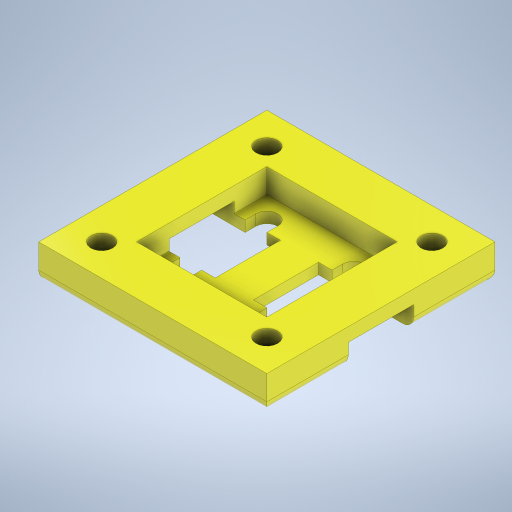
# Autodesk Inventor part: encoder_cover
Saved by Autodesk Inventor 2024 (Build 280153000, 153)
## iProperties
Created: 2021-10-17
Part Number: encoder_cover
Material: Generic
Document SubType Name: Modeling
Designer: jcgg2
Mass: 11.3449 g
Surface Area: 82.1762 cm^2
Volume: 11.3449 cm^3
Density: 1 g/cm^3
Appearance: Yellow
Author: jcgg2
Autodesk Inventor part; units mm, degrees
sketch "Sketch1" plane through (0, 0, 0) normal (0, 1, 0) x (-1, 0, 0)
  line L0 (21, 21) -> (-21, 21)
  line L1 (-21, 21) -> (-21, -21)
  line L2 (-21, -21) -> (21, -21)
  line L3 (21, -21) -> (21, 21)
  line L4 (21, 21) -> (-21, -21) construction
  line L5 (-21, 21) -> (21, -21) construction
  point P0 (0, 0)
  dimension "d0" = 42
  dimension "d1" = 42
  constraints: 12 end point, 2 midpoint, 2 parallel, 1 horizontal, 1 perpendicular
  measures "d0" distance of L2.end L1.end
  measures "d1" distance of L1.end L0.end
extrude "Extrusion1" add sketch "Sketch1" along normal blind 6.5
sketch "Sketch2" plane through (0, 6.5, 0) normal (0, 1, 0) x (1, 0, 0)
  line L0 (-12, -12) -> (12, -12)
  line L1 (12, -12) -> (12, 12)
  line L2 (12, 12) -> (-12, 12)
  line L3 (-12, 12) -> (-12, -12)
  line L4 (-12, -12) -> (12, 12) construction
  line L5 (12, -12) -> (-12, 12) construction
  point P0 (0, 0)
  dimension "d4" = 24
  dimension "d5" = 24
  constraints: 12 end point, 2 midpoint, 2 parallel, 1 horizontal, 1 perpendicular
  measures "d4" distance of L2.end L1.end
  measures "d5" distance of L1.end L0.end
extrude "Extrusion2" cut sketch "Sketch2" against normal blind 4.5
sketch "Sketch3" plane through (0, 2, 0) normal (0, 1, 0) x (1, 0, 0)
  line L0 (-10.5, -6) -> (-3.5, -6)
  line L1 (-3.5, -6) -> (-3.5, 6)
  line L2 (-3.5, 6) -> (-10.5, 6)
  line L3 (-10.5, 6) -> (-10.5, -6)
  line L4 (-10.5, -6) -> (-3.5, 6) construction
  line L5 (-3.5, -6) -> (-10.5, 6) construction
  line L6 (-12, -12) -> (-12, 12) projected
  line L7 (3.5, -6) -> (10.5, -6)
  line L8 (10.5, -6) -> (10.5, 6)
  line L9 (10.5, 6) -> (3.5, 6)
  line L10 (3.5, 6) -> (3.5, -6)
  line L11 (3.5, -6) -> (10.5, 6) construction
  line L12 (10.5, -6) -> (3.5, 6) construction
  line L13 (12, 12) -> (12, -12) projected
  point P0 (0, 0)
  point P1 (-7, 0)
  point P2 (-7, 0)
  point P3 (7, 0)
  point P4 (7, 0)
  dimension "d8" = 7
  dimension "d9" = 12
  dimension "d10" = 1.5
  dimension "d11" = 7
  dimension "d12" = 1.5
  dimension "d13" = 12
  constraints: 24 end point, 6 midpoint, 4 parallel, 2 horizontal, 2 horizontal alignment, 2 perpendicular
  measures "d8" distance of L2.end L1.end
  measures "d9" distance of L1.end L0.end
  measures "d10" distance between parallel lines of L6 L3
  measures "d11" distance of L9.end L8.end
  measures "d12" distance between parallel lines of L8 L13
  measures "d13" distance of L7.end L8.end
extrude "Extrusion3" cut sketch "Sketch3" against normal blind 3.5
sketch "Sketch4" plane through (0, 2, 0) normal (0, 1, 0) x (1, 0, 0)
  line L0 (-12, -12) -> (-12, 12) projected
  line L1 (12, -12) -> (-12, -12) projected
  point P0 (0, 0)
  point P1 (-8, -8)
  point P2 (-8, 8)
  point P3 (8, 8)
  point P4 (8, -8)
  dimension "d16" = 16
  dimension "d17" = 16
  dimension "d18" = 4
  dimension "d19" = 4
  constraints: 2 horizontal alignment, 2 vertical alignment
  measures "d16" distance of point (-8, -8) point (-8, 8)
  measures "d17" distance of point (-8, -8) point (8, -8)
  measures "d18" distance from line of L0 point (-8, -8)
  measures "d19" distance from line of L1 point (-8, -8)
hole "Hole1" at (-8, 2, 8) at (-8, 2, -8) at (8, 2, -8) at (8, 2, 8) direction (0, -1, 0) diameter 4 end through all
sketch "Sketch5" plane through (0, 6.5, 0) normal (0, 1, 0) x (1, 0, 0)
  line L0 (-21, -21) -> (21, -21) projected
  line L1 (-21, 21) -> (-21, -21) projected
  point P0 (0, 0)
  point P1 (-15.2, -15.2)
  point P2 (-15.2, 15.2)
  point P3 (15.2, 15.2)
  point P4 (15.2, -15.2)
  dimension "d27" = 30.4
  dimension "d28" = 30.4
  dimension "d29" = 5.8
  dimension "d30" = 5.8
  constraints: 2 horizontal alignment, 2 vertical alignment
  measures "d27" distance of point (-15.2, 15.2) point (-15.2, -15.2)
  measures "d28" distance of point (15.2, -15.2) point (-15.2, -15.2)
  measures "d29" distance from line of L0 point (-15.2, -15.2)
  measures "d30" distance from line of L1 point (-15.2, -15.2)
hole "Hole2" at (-15.2, 6.5, 15.2) at (-15.2, 6.5, -15.2) at (15.2, 6.5, -15.2) at (15.2, 6.5, 15.2) direction (0, -1, 0) diameter 4 end through all
ref_plane "Work Plane5" through (-25, 0, -21) normal (-1, 0, 0) x (0, 0, 1)
sketch "Sketch9" plane through (-25, 0, -21) normal (-1, 0, 0) x (0, 0, 1)
  point P0 (21, 0)
ref_plane "Work Plane4" through (25, 0, 21) normal (1, 0, 0) x (0, 0, -1)
sketch "Sketch10" plane through (25, 0, 21) normal (1, 0, 0) x (0, 0, -1)
  line L0 (27, 2) -> (31, 2) projected
  line L1 (27, 2) -> (15, 2) projected
  line L2 (11, 2) -> (15, 2) projected
  line L3 (15, 2) -> (27, 2) projected
  line L4 (27, 2) -> (31, 2) projected
  line L5 (27, 2) -> (15, 2) projected
  line L6 (11, 2) -> (15, 2) projected
  line L7 (15, 2) -> (27, 2) projected
  line L8 (33, 2) -> (9, 2) projected
  line L9 (9, 2) -> (33, 2) projected
  line L10 (27, 2) -> (15, 2) projected
  line L11 (27, 2) -> (27, 0) projected
  line L12 (15, 2) -> (27, 2) projected
  line L13 (15, 2) -> (15, 0) projected
  line L14 (27, 0) -> (15, 0) projected
  point P0 (21, 0)
  constraints: 1 other
extrude "Extrusion7" cut sketch "Sketch10" against normal blind 15
ref_plane "Work Plane6" through (-25, 0, -21) normal (-1, 0, 0) x (0, 0, 1)
sketch "Sketch11" plane through (-25, 0, -21) normal (-1, 0, 0) x (0, 0, 1)
  line L0 (27, 2) -> (27, 0) projected
  line L1 (15, 2) -> (27, 2) projected
  line L2 (15, 2) -> (15, 0) projected
  line L3 (27, 0) -> (15, 0) projected
  point P0 (21, 0)
extrude "Extrusion8" cut sketch "Sketch11" against normal blind 15
ref_plane "Work Plane7" through (-25, 0, 6) normal (-1, 0, 0) x (0, 0, 1)
ref_plane "Work Plane8" through (-25, 0, 6) normal (-1, 0, 0) x (0, 0, 1)
ref_plane "Work Plane9" through (-25, 2, -6) normal (0, -1, 0) x (1, 0, 0)
sketch "Sketch16" plane through (-25, 2, -6) normal (0, -1, 0) x (1, 0, 0)
  line L0 (13, 12) -> (13, 0) projected
  line L1 (4, 12) -> (13, 12) projected
  line L2 (4, 0) -> (13, 0) projected
  line L3 (37, 0) -> (37, 12) projected
  line L4 (50, 0) -> (37, 0) projected
  line L5 (50, 12) -> (50, 0) projected
  line L6 (50, 12) -> (37, 12) projected
  line L7 (4, 0) -> (4, 12) projected
  point P0 (25, 6)
extrude "Extrusion11" cut sketch "Sketch16" against normal blind 2
ref_plane "Work Plane10" through (-21, 6.5, 21) normal (1, 0, 0) x (0, 0, -1)
ref_plane "Work Plane11" through (-25, 0, 6) normal (-1, 0, 0) x (0, 0, 1)
fillet "Fillet4" radius 2 4 edges at (21, 0, -13.5) (21, 0, 13.5) (0, 0, -21) (0, 0, 21)
ref_plane "Work Plane12" through (-21.8, 6.5, 21) normal (1, 0, 0) x (0, 0, -1)
sketch "Sketch21" plane through (0, 0, 0) normal (0, -1, 0) x (1, 0, 0)
  circle A0 centre (8, 8) radius 2 projected
  circle A1 centre (8, -8) radius 2 projected
  circle A2 centre (-8, -8) radius 2 projected
  circle A3 centre (-8, 8) radius 2 projected
  circle A4 centre (-8, 8) radius 2 projected
  line L0 (-10, 8) -> (-6, 8)
  line L1 (-6, 8) -> (-6, -8)
  line L2 (-6, -8) -> (-10, -8)
  line L3 (-10, -8) -> (-10, 8)
  line L4 (6, 8) -> (10, 8)
  line L5 (10, 8) -> (10, -8)
  line L6 (10, -8) -> (6, -8)
  line L7 (6, -8) -> (6, 8)
  point P0 (0, 0)
  point P1 (8, 6)
  point P2 (8, -6)
  point P3 (-8, -6)
  point P4 (-8, 6)
  point P5 (10, 8)
  point P6 (-6, 8)
  constraints: 16 end point, 4 parallel, 4 point on circle, 2 horizontal, 2 midpoint, 2 perpendicular, 2 point on line, 1 other
extrude "Extrusion16" cut sketch "Sketch21" against normal blind 3 contours L5 A1 L7 A0 | A2 L3 A3 L1
body "Solid1"
